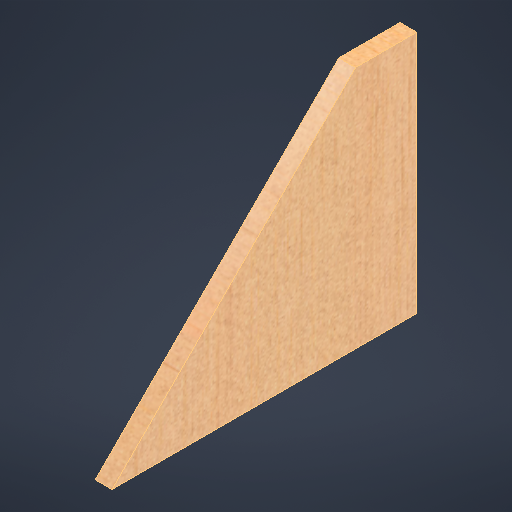
# Autodesk Inventor part: turret_lift
Saved by Autodesk Inventor 2026.2 (Build 302298000, 298)
## iProperties
Created: 2026-01-17
Part Number: turret_lift
Material: Pine
Document SubType Name: Modeling
Designer: User
Density: 0.570257 g/cm^3
Appearance: Yellow Pine - Solid Natural Low Gloss
Author: User
Autodesk Inventor part; units mm, degrees
ref_plane "YZ Plane" through (0, 0, 0) normal (1, 0, 0) x (0, 1, 0)
ref_plane "XZ Plane" through (0, 0, 0) normal (0, 1, 0) x (-1, 0, 0)
ref_plane "XY Plane" through (0, 0, 0) normal (0, 0, 1) x (1, 0, 0)
sketch "Sketch1" plane through (0, 0, 0) normal (1, 0, 0) x (0, 1, 0)
  line L0 (0, 0) -> (139.4187, 0)
  line L1 (139.4187, 0) -> (139.4187, 35)
  line L2 (139.4187, 35) -> (0, 35)
  line L3 (0, 35) -> (0, 0)
  line L4 (139.4187, 35) -> (0, 174.4188)
  line L5 (139.4187, 35) -> (336.5866, 35) construction
  line L6 (0, 174.4188) -> (0, 35)
  dimension "d0" = 139.4187
  dimension "d1" = 35
  dimension "d2" = 135
  dimension "d3" = 174.4187
  constraints: 14 end point, 2 horizontal, 2 parallel, 1 equal length, 1 perpendicular, 1 vertical
  measures "d0" distance of L0.start L0.end
  measures "d1" distance of L0.end L1.end
  measures "d2" angle of L5 L4
  measures "d3" distance of L4.end L0.start
extrude "Extrusion1" add sketch "Sketch1" along normal blind 9.5813
body "Solid1"
